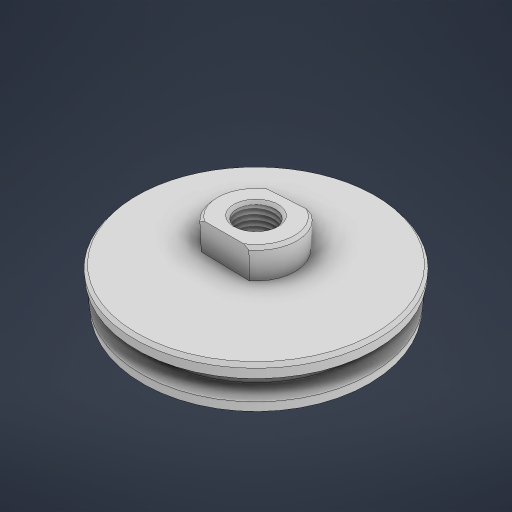
# Autodesk Inventor part: Endcap
Saved by Autodesk Inventor 2024.1 (Build 281209000, 209)
## iProperties
Created: 2023-02-11
Part Number: Endcap
Material: Steel
Document SubType Name: Modeling
Designer: Sven
Density: 7.85 g/cm^3
Appearance: Default
Mass: 80.5949 g
Surface Area: 49.448 cm^2
Volume: 10.2669 cm^3
Author: Sven
Autodesk Inventor part; units mm, degrees
ref_plane "YZ Plane" through (0, 0, 0) normal (1, 0, 0) x (0, 1, 0)
ref_plane "XZ Plane" through (0, 0, 0) normal (0, 1, 0) x (-1, 0, 0)
ref_plane "XY Plane" through (0, 0, 0) normal (0, 0, 1) x (1, 0, 0)
sketch "Sketch6" plane through (0, 0, 0) normal (1, 0, 0) x (0, 1, 0)
  line L0 (0, 0) -> (12.5, 0)
  line L1 (0, 0) -> (0, -21.75)
  line L2 (0, -21.75) -> (2, -21.75)
  line L3 (2, -21.75) -> (2, -18.75)
  line L4 (2, -18.75) -> (5.5, -18.75)
  line L5 (5.5, -18.75) -> (5.5, -21.75)
  line L6 (5.5, -21.75) -> (7.5, -21.75)
  line L7 (7.5, -21.75) -> (7.5, -7)
  line L8 (7.5, -7) -> (12.5, -7)
  line L9 (12.5, -7) -> (12.5, 0)
  point P0 (6.25, 0)
  dimension "d28" = 43.5
  dimension "d29" = 14
  dimension "d30" = 5
  dimension "d31" = 7
  dimension "d33" = 3.5
  dimension "d35" = 12.5
  dimension "d36" = 37.5
  constraints: 20 end point, 7 perpendicular, 2 point on line, 1 horizontal, 1 midpoint, 1 vertical
  measures "d28" diameter of L2 L0
  measures "d29" diameter of L8 point (6.25, 0)
  measures "d30" distance between parallel lines of L7 L9
  measures "d31" distance between parallel lines of L5 L9
  measures "d33" distance between parallel lines of L3 L5
  measures "d35" distance between parallel lines of L1 L9
  measures "d36" diameter of L4 L0
revolve "Revolution3" add sketch "Sketch6" angle 360 about axis through (0, 0, 0) along (0, 1, 0)
hole "Hole2" at (0, 12.5, 0) direction (0, -1, 0) diameter 6.561 end through all thread size "G 1/16-28" standard "BSP Pipe Threads"
sketch "Sketch7" plane through (0, 12.5, 0) normal (0, 1, 0) x (1, 0, 0)
  circle A0 centre (0, 0) radius 7 construction
  line L0 (-4.3301, -5.5) -> (4.3301, -5.5)
  line L1 (7, 0) -> (-7, 0)
  line L2 (-4.3301, 5.5) -> (4.3301, 5.5)
  arc A1 (-4.3301, -5.5) -> (4.3301, -5.5) centre (0, 0) ccw
  arc A2 (4.3301, 5.5) -> (-4.3301, 5.5) centre (0, 0) ccw
  dimension "d49" = 11
  constraints: 8 point on circle, 6 end point, 2 centre point, 2 symmetric about line, 1 coincident, 1 horizontal, 1 midpoint, 1 other
  measures "d49" distance between parallel lines of L2 L0
extrude "Extrusion2" cut sketch "Sketch7" against normal up to surface (5 mm away)
chamfer "Chamfer5" distance 0.5 angle 45 6 edges at (0, 0, 21.75) (0, 7.5, 21.75) (7, 12.5, 0) (-7, 12.5, 0) (0, 0, -3.2805) (0, 12.5, -3.2805)
body "Solid2"
